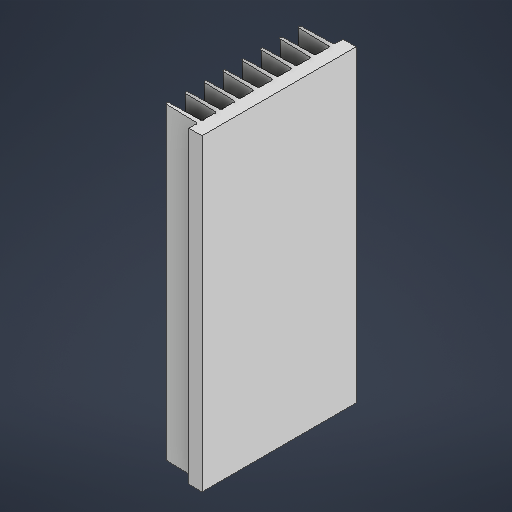
# Autodesk Inventor part: HeatSink3.5-7in stock
Saved by Autodesk Inventor 2026.1 (Build 301233020, 233B)
## iProperties
Created: 2025-09-11
Part Number: HeatSink3.5-7in stock
Material: Generic
Document SubType Name: Modeling
Designer: atrus
Density: 1 g/cm^3
Appearance: Default
Author: atrus
Autodesk Inventor part; units mm, degrees
ref_plane "YZ Plane" through (0, 0, 0) normal (1, 0, 0) x (0, 1, 0)
ref_plane "XZ Plane" through (0, 0, 0) normal (0, 1, 0) x (-1, 0, 0)
ref_plane "XY Plane" through (0, 0, 0) normal (0, 0, 1) x (1, 0, 0)
sketch "Sketch1" plane through (0, 0, 0) normal (0, 1, 0) x (-1, 0, 0)
  line L0 (0, 0) -> (0, -88.9)
  line L1 (0, -88.9) -> (7.62, -88.9)
  line L2 (7.62, -88.9) -> (7.62, -85.7877)
  line L3 (0, 0) -> (7.62, 0)
  line L4 (7.62, 0) -> (7.62, -4.2675)
  line L5 (8.3611, -5.0292) -> (25.9289, -5.5121)
  line L6 (25.9289, -7.0355) -> (8.3611, -7.5184)
  line L7 (7.62, -8.2801) -> (7.62, -15.1641)
  line L8 (8.3611, -15.9258) -> (25.9289, -16.4087)
  line L9 (25.9289, -17.9321) -> (8.3611, -18.415)
  line L10 (7.62, -19.1767) -> (7.62, -26.0607)
  line L11 (8.3611, -26.8224) -> (25.9289, -27.3053)
  line L12 (25.9289, -28.8287) -> (8.3611, -29.3116)
  line L13 (7.62, -30.0733) -> (7.62, -36.9573)
  line L14 (8.3611, -37.719) -> (25.9289, -38.2019)
  line L15 (25.9289, -39.7253) -> (8.3611, -40.2082)
  line L16 (7.62, -85.7877) -> (7.62, -84.5563)
  line L17 (8.3611, -83.7946) -> (25.9289, -83.3117)
  line L18 (25.9289, -81.7883) -> (8.3611, -81.3054)
  line L19 (7.62, -80.5437) -> (7.62, -73.6597)
  line L20 (8.3611, -72.898) -> (25.9289, -72.4151)
  line L21 (25.9289, -70.8917) -> (8.3611, -70.4088)
  line L22 (7.62, -69.6471) -> (7.62, -62.7631)
  line L23 (8.3611, -62.0014) -> (25.9289, -61.5185)
  line L24 (25.9289, -59.9951) -> (8.3611, -59.5122)
  line L25 (7.62, -58.7505) -> (7.62, -51.8665)
  line L26 (7.62, -40.9699) -> (7.62, -47.8539)
  line L27 (8.3611, -48.6156) -> (25.9289, -49.0985)
  line L28 (25.9289, -50.6219) -> (8.3611, -51.1048)
  arc A0 (25.9289, -7.0355) -> (25.9289, -5.5121) centre (25.908, -6.2738) ccw
  arc A1 (25.9289, -17.9321) -> (25.9289, -16.4087) centre (25.908, -17.1704) ccw
  arc A2 (25.9289, -28.8287) -> (25.9289, -27.3053) centre (25.908, -28.067) ccw
  arc A3 (25.9289, -39.7253) -> (25.9289, -38.2019) centre (25.908, -38.9636) ccw
  arc A4 (25.9289, -50.6219) -> (25.9289, -49.0985) centre (25.908, -49.8602) ccw
  arc A5 (25.9289, -61.5185) -> (25.9289, -59.9951) centre (25.908, -60.7568) ccw
  arc A6 (25.9289, -72.4151) -> (25.9289, -70.8917) centre (25.908, -71.6534) ccw
  arc A7 (25.9289, -83.3117) -> (25.9289, -81.7883) centre (25.908, -82.55) ccw
  arc A8 (7.62, -4.2675) -> (8.3611, -5.0292) centre (8.382, -4.2675) ccw
  arc A9 (8.3611, -7.5184) -> (7.62, -8.2801) centre (8.382, -8.2801) ccw
  arc A10 (7.62, -15.1641) -> (8.3611, -15.9258) centre (8.382, -15.1641) ccw
  arc A11 (8.3611, -18.415) -> (7.62, -19.1767) centre (8.382, -19.1767) ccw
  arc A12 (7.62, -26.0607) -> (8.3611, -26.8224) centre (8.382, -26.0607) ccw
  arc A13 (8.3611, -29.3116) -> (7.62, -30.0733) centre (8.382, -30.0733) ccw
  arc A14 (7.62, -36.9573) -> (8.3611, -37.719) centre (8.382, -36.9573) ccw
  arc A15 (8.3611, -40.2082) -> (7.62, -40.9699) centre (8.382, -40.9699) ccw
  arc A16 (7.62, -47.8539) -> (8.3611, -48.6156) centre (8.382, -47.8539) ccw
  arc A17 (8.3611, -51.1048) -> (7.62, -51.8665) centre (8.382, -51.8665) ccw
  arc A18 (7.62, -58.7505) -> (8.3611, -59.5122) centre (8.382, -58.7505) ccw
  arc A19 (8.3611, -62.0014) -> (7.62, -62.7631) centre (8.382, -62.7631) ccw
  arc A20 (7.62, -69.6471) -> (8.3611, -70.4088) centre (8.382, -69.6471) ccw
  arc A21 (8.3611, -72.898) -> (7.62, -73.6597) centre (8.382, -73.6597) ccw
  arc A22 (7.62, -80.5437) -> (8.3611, -81.3054) centre (8.382, -80.5437) ccw
  arc A23 (8.3611, -83.7946) -> (7.62, -84.5563) centre (8.382, -84.5563) ccw
  point P0 (7.62, -7.5388)
  point P1 (7.62, -15.9054)
  point P2 (7.62, -18.4354)
  point P3 (7.62, -26.802)
  point P4 (7.62, -29.332)
  point P5 (7.62, -37.6986)
  point P6 (7.62, -40.2286)
  point P7 (7.62, -81.285)
  point P8 (7.62, -72.9184)
  point P9 (7.62, -70.3884)
  point P10 (7.62, -62.0218)
  point P11 (7.62, -59.4918)
  point P12 (7.62, -51.1252)
  point P13 (26.67, -82.55)
  point P14 (3.81, -88.9)
  dimension "d0" = 88.9
  dimension "d1" = 7.62
  dimension "d3" = 0.762
  dimension "d4" = 0.762
  dimension "d5" = 0.762
  dimension "d6" = 26.67
  dimension "d8" = 2.4892
  dimension "d9" = 6.35
  dimension "d10" = 10.8966
  constraints: 58 end point, 49 point on circle, 48 tangent, 38 point on line, 24 centre point, 21 equal radius, 14 parallel, 8 equal length, 8 vertical alignment, 3 vertical, 2 perpendicular, 1 collinear, 1 horizontal, 1 midpoint
  measures "d0" distance of L0.start L0.end
  measures "d1" distance of L0.end L1.end
  measures "d3" radius of A0
  measures "d4" radius of A8
  measures "d5" radius of A15
  measures "d6" horizontal distance of L0.end point (26.67, -82.55)
  measures "d8" distance of L6.end L5.start
  measures "d9" vertical distance of point (3.81, -88.9) A7.centre
  measures "d10" distance of A1.centre A0.centre
extrude "Extrusion1" add sketch "Sketch1" along normal blind 177.8
body "Solid1"
